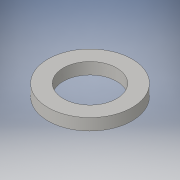
# Autodesk Inventor part: vexSupportRing
Saved by Autodesk Inventor 2016 SP1 (Build 200210100, 210)
## iProperties
Created: 2015-11-19
Part Number: vexSupportRing
Material: Generic
Document SubType Name: Modeling
Designer: steele
Density: 1 g/cm^3
Appearance: Default
Author: steele
Autodesk Inventor part; units mm, degrees
ref_plane "YZ Plane" through (0, 0, 0) normal (1, 0, 0) x (0, 1, 0)
ref_plane "XZ Plane" through (0, 0, 0) normal (0, 1, 0) x (-1, 0, 0)
ref_plane "XY Plane" through (0, 0, 0) normal (0, 0, 1) x (1, 0, 0)
sketch "Sketch1" plane through (0, 0, 0) normal (0, 1, 0) x (-1, 0, 0)
  circle A0 centre (0, 0) radius 51.5874
  circle A1 centre (0, 0) radius 81.2419
  dimension "d0" = 103.1748
  dimension "d1" = 162.4838
  constraints: 2 centre point, 2 coincident
  measures "d0" diameter of A0
  measures "d1" diameter of A1
extrude "Extrusion1" add sketch "Sketch1" along normal blind 22.479
equation "\"d0\" = insideDiam"
equation "\"d1\" = outsideDiam"
equation "\"d2\" = thickness"
equation "\"thickness\" = 22.479"
equation "\"printerError\" = 0.508"
equation "\"insideDiam\" = 103.1748"
equation "\"outsideDiam\" = 162.4838"
body "Solid1"
